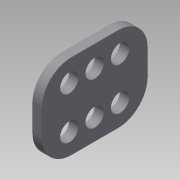
# Autodesk Inventor part: BottomToBottom
Saved by Autodesk Inventor 2014 (Build 180170000, 170)
## iProperties
Created: 2014-03-07
Part Number: BottomToBottom
Material: Générique
Document SubType Name: Modeling
Designer: Grégoire
Density: 1 g/cm^3
Appearance: Par défaut
Author: Grégoire
Autodesk Inventor part; units mm, degrees
ref_plane "YZ Plane" through (0, 0, 0) normal (1, 0, 0) x (0, 1, 0)
ref_plane "XZ Plane" through (0, 0, 0) normal (0, 1, 0) x (-1, 0, 0)
ref_plane "XY Plane" through (0, 0, 0) normal (0, 0, 1) x (1, 0, 0)
sketch "Esquisse11" plane through (0, 0, 0) normal (1, 0, 0) x (0, 1, 0)
  line L0 (0, 0) -> (25, 0)
  line L1 (25, 0) -> (25, 10)
  line L2 (25, 10) -> (0, 10)
  line L3 (0, 10) -> (0, 0)
  line L4 (12.5, 0) -> (12.5, 10) construction
  circle A0 centre (12.5, 5) radius 2.15
  line L5 (12.5, 5) -> (25, 5) construction
  circle A1 centre (18.5, 5) radius 2.15
  circle A2 centre (6.5, 5) radius 2.15
  circle A3 centre (12.5, 5) radius 2.15
  dimension "d118" = 25
  dimension "d119" = 10
  dimension "d120" = 5
  dimension "d121" = 4.3
  dimension "d124" = 6
  dimension "d127" = 6
  constraints: 12 end point, 4 centre point, 4 midpoint, 3 horizontal, 2 parallel, 2 perpendicular, 6 other
  measures "d118" distance of L0.start L0.end
  measures "d119" distance of L2.end L0.start
  measures "d120" distance from line of L0 L5.start
  measures "d121" diameter of A0
  measures "d124" distance of L5.start A1.centre
  measures "d127" distance of L5.start A2.centre
extrude "Extrusion11" add sketch "Esquisse11" along normal blind 2.2
fillet "Congé7" radius 7 2 edges at (1.1, 0, 0) (1.1, 25, 0)
mirror "Symétrie2" about plane through (0, 25, 10) normal (0, 0, 1)
equation "\"d121\" = Holes"
equation "\"d130\" = Depth"
equation "\"d132\" = Rounding"
equation "\"Depth\" = 2.2"
equation "\"Holes\" = 4.3"
equation "\"Height\" = 0"
equation "\"Rounding\" = 7"
